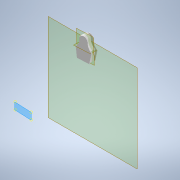
# Autodesk Inventor part: sprocket7_mk2_tips
Saved by Autodesk Inventor 2020 (Build 240168000, 168)
## iProperties
Created: 2019-08-05
Part Number: sprocket7_mk2_tips
Material: Generic
Document SubType Name: Modeling
Designer: erwin
Density: 1 g/cm^3
Appearance: Default
Author: erwin
Autodesk Inventor part; units mm, degrees
ref_plane "YZ Plane" through (0, 0, 0) normal (1, 0, 0) x (0, 1, 0)
ref_plane "XZ Plane" through (0, 0, 0) normal (0, 1, 0) x (-1, 0, 0)
ref_plane "XY Plane" through (0, 0, 0) normal (0, 0, 1) x (1, 0, 0)
ref_plane "Work Plane1" through (6.098, -2.6064, -12) normal (0, 0, -1) x (-1, 0, 0)
sketch "Sketch1" plane through (6.098, -2.6064, -12) normal (0, 0, -1) x (-1, 0, 0)
  circle A0 centre (7.1179, -1.5237) radius 10.75 construction
  arc A1 (21.9255, 105.301) -> (1.9456, 106.1983) centre (11.9355, 105.7496) ccw construction
  line L0 (-93.2965, -27.178) -> (-90.244, -26.8147) projected
  line L1 (-90.244, -26.8147) -> (-85.3551, -26.6226) projected
  line L2 (-85.3551, -26.6226) -> (-80.6041, -27.7915) projected
  line L3 (-80.6041, -27.7915) -> (-76.3624, -30.2299) projected
  line L4 (-76.3624, -30.2299) -> (-72.9614, -33.7473) projected
  line L5 (-72.9614, -33.7473) -> (-48.2745, -67.726) projected
  line L6 (-48.2745, -67.726) -> (-45.9802, -72.0474) projected
  line L7 (-45.9802, -72.0474) -> (-44.9719, -76.835) projected
  line L8 (-44.9719, -76.835) -> (-45.3284, -81.7147) projected
  line L9 (-45.3284, -81.7147) -> (-47.0218, -86.3049) projected
  line L10 (-47.0218, -86.3049) -> (-48.3106, -89.0958) projected
  line L11 (-48.3106, -89.0958) -> (-48.988, -90.8804) projected
  line L12 (-48.988, -90.8804) -> (-49.1805, -92.7796) projected
  line L13 (-49.1805, -92.7796) -> (-48.8748, -94.6639) projected
  line L14 (-48.8748, -94.6639) -> (-48.0919, -96.4049) projected
  line L15 (-48.0919, -96.4049) -> (-46.885, -97.8839) projected
  line L16 (-46.885, -97.8839) -> (-45.3365, -99.0002) projected
  line L17 (-45.3365, -99.0002) -> (-43.5518, -99.6776) projected
  line L18 (-43.5518, -99.6776) -> (-41.6526, -99.87) projected
  line L19 (-41.6526, -99.87) -> (-39.7683, -99.5643) projected
  line L20 (-39.7683, -99.5643) -> (-38.0273, -98.7814) projected
  line L21 (-38.0273, -98.7814) -> (-36.5483, -97.5745) projected
  line L22 (-36.5483, -97.5745) -> (-35.4321, -96.026) projected
  line L23 (-35.4321, -96.026) -> (-33.8129, -93.4129) projected
  line L24 (-33.8129, -93.4129) -> (-30.9149, -89.4709) projected
  line L25 (-30.9149, -89.4709) -> (-27.0389, -86.4852) projected
  line L26 (-27.0389, -86.4852) -> (-22.4878, -84.6892) projected
  line L27 (-22.4878, -84.6892) -> (-17.6173, -84.2233) projected
  line L28 (-17.6173, -84.2233) -> (24.3404, -86.1076) projected
  line L29 (24.3404, -86.1076) -> (29.1494, -87.0082) projected
  line L30 (29.1494, -87.0082) -> (33.5212, -89.2049) projected
  line L31 (33.5212, -89.2049) -> (37.114, -92.5261) projected
  line L32 (37.114, -92.5261) -> (39.647, -96.712) projected
  line L33 (39.647, -96.712) -> (41.0254, -99.4597) projected
  line L34 (41.0254, -99.4597) -> (41.9983, -101.1021) projected
  line L35 (41.9983, -101.1021) -> (43.3632, -102.4367) projected
  line L36 (43.3632, -102.4367) -> (45.027, -103.3725) projected
  line L37 (45.027, -103.3725) -> (46.8763, -103.8459) projected
  line L38 (46.8763, -103.8459) -> (48.7851, -103.8244) projected
  line L39 (48.7851, -103.8244) -> (50.6233, -103.3097) projected
  line L40 (50.6233, -103.3097) -> (52.2657, -102.3368) projected
  line L41 (52.2657, -102.3368) -> (53.6003, -100.9719) projected
  line L42 (53.6003, -100.9719) -> (54.5361, -99.3081) projected
  line L43 (54.5361, -99.3081) -> (55.0095, -97.4588) projected
  line L44 (55.0095, -97.4588) -> (54.988, -95.55) projected
  line L45 (54.988, -95.55) -> (54.4733, -93.7118) projected
  line L46 (54.4733, -93.7118) -> (53.4399, -90.8167) projected
  line L47 (53.4399, -90.8167) -> (52.1647, -86.0931) projected
  line L48 (52.1647, -86.0931) -> (52.2471, -81.2011) projected
  line L49 (52.2471, -81.2011) -> (53.6805, -76.5231) projected
  line L50 (53.6805, -76.5231) -> (56.3529, -72.4248) projected
  line L51 (56.3529, -72.4248) -> (83.9863, -40.7958) projected
  line L52 (83.9863, -40.7958) -> (87.6888, -37.5974) projected
  line L53 (87.6888, -37.5974) -> (92.1321, -35.5491) projected
  line L54 (92.1321, -35.5491) -> (96.9687, -34.8108) projected
  line L55 (96.9687, -34.8108) -> (101.8207, -35.4404) projected
  line L56 (101.8207, -35.4404) -> (104.8283, -36.0758) projected
  line L57 (104.8283, -36.0758) -> (106.719, -36.3391) projected
  line L58 (106.719, -36.3391) -> (108.6134, -36.1041) projected
  line L59 (108.6134, -36.1041) -> (110.3825, -35.3868) projected
  line L60 (110.3825, -35.3868) -> (111.9056, -34.2361) projected
  line L61 (111.9056, -34.2361) -> (113.0789, -32.7304) projected
  line L62 (113.0789, -32.7304) -> (113.8226, -30.9723) projected
  line L63 (113.8226, -30.9723) -> (114.0859, -29.0816) projected
  line L64 (114.0859, -29.0816) -> (113.8509, -27.1872) projected
  line L65 (113.8509, -27.1872) -> (113.1336, -25.4182) projected
  line L66 (113.1336, -25.4182) -> (111.9829, -23.8951) projected
  line L67 (111.9829, -23.8951) -> (110.4772, -22.7217) projected
  line L68 (110.4772, -22.7217) -> (108.7191, -21.978) projected
  line L69 (108.7191, -21.978) -> (105.8112, -20.9809) projected
  line L70 (105.8112, -20.9809) -> (101.3232, -19.0328) projected
  line L71 (101.3232, -19.0328) -> (97.5498, -15.9183) projected
  line L72 (97.5498, -15.9183) -> (94.7861, -11.881) projected
  line L73 (94.7861, -11.881) -> (93.2481, -7.2363) projected
  line L74 (93.2481, -7.2363) -> (85.7487, 34.0887) projected
  line L75 (85.7487, 34.0887) -> (85.5567, 38.9776) projected
  line L76 (85.5567, 38.9776) -> (86.7255, 43.7286) projected
  line L77 (86.7255, 43.7286) -> (89.1639, 47.9703) projected
  line L78 (89.1639, 47.9703) -> (92.6813, 51.3713) projected
  line L79 (92.6813, 51.3713) -> (95.0533, 53.3265) projected
  line L80 (95.0533, 53.3265) -> (96.438, 54.6406) projected
  line L81 (96.438, 54.6406) -> (97.4354, 56.2682) projected
  line L82 (97.4354, 56.2682) -> (97.9776, 58.0985) projected
  line L83 (97.9776, 58.0985) -> (98.0276, 60.0068) projected
  line L84 (98.0276, 60.0068) -> (97.5819, 61.8629) projected
  line L85 (97.5819, 61.8629) -> (96.6711, 63.5405) projected
  line L86 (96.6711, 63.5405) -> (95.357, 64.9252) projected
  line L87 (95.357, 64.9252) -> (93.7294, 65.9226) projected
  line L88 (93.7294, 65.9226) -> (91.8991, 66.4648) projected
  line L89 (91.8991, 66.4648) -> (89.9908, 66.5148) projected
  line L90 (89.9908, 66.5148) -> (88.1347, 66.0691) projected
  line L91 (88.1347, 66.0691) -> (86.4571, 65.1583) projected
  line L92 (86.4571, 65.1583) -> (83.8645, 63.5065) projected
  line L93 (83.8645, 63.5065) -> (79.5431, 61.2122) projected
  line L94 (79.5431, 61.2122) -> (74.7554, 60.204) projected
  line L95 (74.7554, 60.204) -> (69.8758, 60.5605) projected
  line L96 (69.8758, 60.5605) -> (65.2855, 62.2539) projected
  line L97 (65.2855, 62.2539) -> (28.3005, 82.1564) projected
  line L98 (28.3005, 82.1564) -> (24.3585, 85.0544) projected
  line L99 (24.3585, 85.0544) -> (21.3728, 88.9304) projected
  line L100 (21.3728, 88.9304) -> (19.5768, 93.4815) construction
  line L101 (19.5768, 93.4815) -> (19.1109, 98.3519) projected
  line L102 (19.1109, 98.3519) -> (19.0611, 101.4256) projected
  line L103 (19.0611, 101.4256) -> (18.8971, 103.3274) projected
  line L104 (18.8971, 103.3274) -> (18.2465, 105.1221) projected
  line L105 (18.2465, 105.1221) -> (17.1535, 106.6871) projected
  line L106 (17.1535, 106.6871) -> (15.6927, 107.916) projected
  line L107 (15.6927, 107.916) -> (13.9636, 108.7249) projected
  line L108 (13.9636, 108.7249) -> (12.0841, 109.0587) projected
  line L109 (12.0841, 109.0587) -> (10.1823, 108.8947) projected
  line L110 (10.1823, 108.8947) -> (8.3877, 108.244) projected
  line L111 (8.3877, 108.244) -> (6.8226, 107.1511) projected
  line L112 (6.8226, 107.1511) -> (5.5937, 105.6903) projected
  line L113 (5.5937, 105.6903) -> (4.7848, 103.9612) projected
  line L114 (4.7848, 103.9612) -> (4.451, 102.0817) projected
  line L115 (4.451, 102.0817) -> (4.126, 99.0249) projected
  line L116 (4.126, 99.0249) -> (3.2253, 94.2159) projected
  line L117 (3.2253, 94.2159) -> (1.0286, 89.8441) construction
  line L118 (1.0286, 89.8441) -> (-2.2925, 86.2513) projected
  line L119 (-2.2925, 86.2513) -> (-6.4785, 83.7183) projected
  line L120 (-6.4785, 83.7183) -> (-45.0987, 67.2113) projected
  line L121 (-45.0987, 67.2113) -> (-49.8222, 65.9361) projected
  line L122 (-49.8222, 65.9361) -> (-54.7142, 66.0184) projected
  line L123 (-54.7142, 66.0184) -> (-59.3922, 67.4518) projected
  line L124 (-59.3922, 67.4518) -> (-63.4905, 70.1242) projected
  line L125 (-63.4905, 70.1242) -> (-65.9246, 72.0017) projected
  line L126 (-65.9246, 72.0017) -> (-67.5138, 73.0593) projected
  line L127 (-67.5138, 73.0593) -> (-69.3226, 73.6695) projected
  line L128 (-69.3226, 73.6695) -> (-71.2276, 73.7908) projected
  line L129 (-71.2276, 73.7908) -> (-73.0992, 73.4149) projected
  line L130 (-73.0992, 73.4149) -> (-74.8096, 72.5674) projected
  line L131 (-74.8096, 72.5674) -> (-76.2425, 71.3061) projected
  line L132 (-76.2425, 71.3061) -> (-77.3001, 69.7169) projected
  line L133 (-77.3001, 69.7169) -> (-77.9103, 67.9081) projected
  line L134 (-77.9103, 67.9081) -> (-78.0316, 66.0031) projected
  line L135 (-78.0316, 66.0031) -> (-77.6557, 64.1315) projected
  line L136 (-77.6557, 64.1315) -> (-76.8082, 62.4211) projected
  line L137 (-76.8082, 62.4211) -> (-75.5468, 60.9882) projected
  line L138 (-75.5468, 60.9882) -> (-73.3596, 58.8282) projected
  line L139 (-73.3596, 58.8282) -> (-70.1612, 55.1256) projected
  line L140 (-70.1612, 55.1256) -> (-68.1129, 50.6824) projected
  line L141 (-68.1129, 50.6824) -> (-67.3746, 45.8458) projected
  line L142 (-67.3746, 45.8458) -> (-68.0042, 40.9938) projected
  line L143 (-68.0042, 40.9938) -> (-79.1777, 0.5073) projected
  line L144 (-79.1777, 0.5073) -> (-81.1259, -3.9807) projected
  line L145 (-81.1259, -3.9807) -> (-84.2403, -7.7541) projected
  line L146 (-84.2403, -7.7541) -> (-88.2777, -10.5178) projected
  line L147 (-88.2777, -10.5178) -> (-92.9223, -12.0558) projected
  line L148 (-92.9223, -12.0558) -> (-95.9078, -12.7882) projected
  line L149 (-95.9078, -12.7882) -> (-97.7255, -13.3713) projected
  line L150 (-97.7255, -13.3713) -> (-99.3304, -14.405) projected
  line L151 (-99.3304, -14.405) -> (-100.613, -15.8188) projected
  line L152 (-100.613, -15.8188) -> (-101.486, -17.5164) projected
  line L153 (-101.486, -17.5164) -> (-101.8898, -19.3821) projected
  line L154 (-101.8898, -19.3821) -> (-101.7971, -21.2888) projected
  line L155 (-101.7971, -21.2888) -> (-101.214, -23.1065) projected
  line L156 (-101.214, -23.1065) -> (-100.1803, -24.7113) projected
  line L157 (-100.1803, -24.7113) -> (-98.7665, -25.9939) projected
  line L158 (-98.7665, -25.9939) -> (-97.0689, -26.8669) projected
  line L159 (-97.0689, -26.8669) -> (-95.2031, -27.2708) projected
  line L160 (-95.2031, -27.2708) -> (-93.2965, -27.178) projected
  circle A2 centre (7.1179, -1.5237) radius 10.75 projected
  circle A3 centre (11.7561, 101.7537) radius 7.2498
  line L161 (-3.033, 62.3775) -> (22.956, 61.2104) projected
  line L162 (-4.0017, 85.217) -> (-3.033, 62.3775) projected
  line L163 (22.956, 61.2104) -> (25.9681, 83.8711) projected
  arc A4 (-4.0017, 85.217) -> (4.5067, 101.6713) centre (-15.2247, 101.4473) ccw
  line L164 (11.7561, 101.7537) -> (7.1179, -1.5237) construction
  arc A5 (18.9689, 101.0219) -> (25.9681, 83.8711) centre (38.6007, 99.03) ccw
  point P0 (6.098, 2.6064)
  point P1 (11.3971, 93.7617)
  point P2 (21.2089, 89.3457)
  point P3 (1.229, 90.2429)
  point P4 (19.0059, 101.7435)
  point P5 (18.9689, 101.0219)
  constraints: 8 point on circle, 5 tangent, 4 centre point, 2 end point, 2 point on line, 2 symmetric about line, 1 other
extrude "Extrusion1" add sketch "Sketch1" against normal blind 12 contours A4 A3 A5 L163 L161 L162 | A3
sketch "Sketch2" plane through (6.098, -2.6064, 0) normal (0, 0, 1) x (-1, 0, 0)
  line L0 (1.229, 90.2429) -> (21.2089, 89.3456) projected
  line L1 (1.229, 90.2429) -> (0.8688, 82.2225) projected
  arc A0 (0.8688, 82.2225) -> (20.8487, 81.3252) centre (10.8588, 81.7738) ccw projected
  line L2 (20.8487, 81.3252) -> (21.2089, 89.3456) projected
  arc A1 (-1.9524, 82.3492) -> (23.67, 81.1985) centre (10.8588, 81.7738) ccw
  line L3 (-1.9524, 82.3492) -> (-1.4655, 93.1909)
  line L4 (-1.4655, 93.1909) -> (24.1569, 92.0402)
  line L5 (24.1569, 92.0402) -> (23.67, 81.1985)
  circle A2 centre (10.8588, 81.7738) radius 12.8241
  circle A3 centre (10.8588, 81.7738) radius 7.8241
  line L6 (20.8487, 81.3252) -> (21.2089, 89.3456) projected
  arc A4 (21.2089, 89.3456) -> (18.6806, 81.5855) centre (32.905, 81.2431) ccw
  line L7 (10.8588, 81.7738) -> (12.0813, 108.9962) construction
  arc A5 (19.0059, 101.7435) -> (4.5341, 102.3888) centre (11.7561, 101.7537) ccw projected
  arc A6 (3.0515, 82.2874) -> (1.229, 90.2429) centre (-11.1463, 83.2214) ccw
  point P0 (6.098, -2.6064)
  point P1 (1.2053, 89.7149)
  point P2 (-1.9524, 82.3492)
  point P3 (21.1852, 88.8176)
  point P4 (1.229, 90.2429)
  point P5 (1.229, 90.2429)
  point P6 (1.0296, 90.0106)
  point P7 (3.0515, 82.2874)
  point P8 (1.229, 90.2429)
  dimension "d10" = 5
  constraints: 9 point on circle, 8 end point, 4 centre point, 3 symmetric about line, 2 coincident, 8 other
sketch "Sketch3" plane through (-4.7607, 79.1674, -11) normal (0, 0, 1) x (0.9989931, 0.0448647, 0)
  arc A0 (-7.8224, 0.1628) -> (7.8224, 0.1628) centre (0, 0) ccw projected
  arc A1 (-7.8224, 0.1628) -> (-10, 8.0286) centre (-22.0479, 0.4589) ccw projected
  arc A2 (-10, 8.0286) -> (10, 8.0286) centre (0, 0) ccw projected
  arc A3 (10, 8.0286) -> (7.8224, 0.1628) centre (22.0479, 0.4589) ccw projected
  arc A4 (-7.9795, 8.0286) -> (-5.2449, 20.5755) centre (-42.9142, 22.2142) ccw projected
  line L0 (-7.9795, 8.0286) -> (7.9795, 8.0286) projected
  arc A5 (5.245, 20.5722) -> (7.9795, 8.0286) centre (42.9142, 22.2142) ccw projected
  arc A6 (5.245, 20.5722) -> (-5.2449, 20.5755) centre (0, 20.3473) ccw projected
  line L1 (0, 20.3473) -> (0, 0) construction
  line L2 (0, 0) -> (0, -15) construction
  line L3 (-12.8241, 0) -> (-12.8241, -15) construction
  line L4 (12.8241, -15) -> (12.8241, 0) construction
  arc A7 (12.8241, 0) -> (-12.8241, 0) centre (0, 0) ccw construction
  arc A8 (-12.8241, -15) -> (12.8241, -15) centre (0, -15) ccw construction
  arc A9 (-10, 8.0286) -> (10, 8.0286) centre (0, 0) ccw construction
  arc A10 (-7.8224, 0.1628) -> (7.8224, 0.1628) centre (0, 0) ccw construction
  line L5 (0, 0) -> (0, -18.52) construction
  line L6 (-6, -14.0249) -> (-6, -18.52) construction
  line L7 (6, -18.52) -> (6, -14.0249) construction
  arc A11 (6, 0) -> (-6, 0) centre (0, 0) ccw construction
  arc A12 (-6, -18.52) -> (6, -18.52) centre (0, -18.52) ccw construction
  line L8 (6, -18.52) -> (6, -11.3339)
  line L9 (-6, -18.52) -> (-6, -11.3339)
  arc A13 (7.9143, -10.0907) -> (-7.9143, -10.0907) centre (0, 0) ccw
  arc A14 (-6, -18.52) -> (6, -18.52) centre (0, -18.52) ccw
  arc A15 (7.9143, -10.0907) -> (6, -14.0249) centre (11, -14.0249) ccw
  arc A16 (-6, -14.0249) -> (-7.9143, -10.0907) centre (-11, -14.0249) ccw
  point P0 (1.2041, -79.3013)
  point P1 (0, -7.5)
  point P2 (0, -9.26)
  point P3 (6, -14.0249)
  point P4 (7.9143, -10.0907)
  point P5 (-7.9143, -10.0907)
  point P6 (-6, -14.0249)
  dimension "d17" = 15
  dimension "d18" = 12
  dimension "d19" = 5
  constraints: 22 end point, 21 point on circle, 12 tangent, 8 centre point, 5 point on line, 2 coincident, 2 equal radius, 2 midpoint, 2 parallel, 1 collinear, 1 vertical
  measures "d17" distance of L1.end L2.end
  measures "d18" diameter of A12
  measures "d19" radius of A15
sketch "Sketch4" plane through (-4.7607, 79.1674, -11) normal (0, 0, 1) x (0.9989931, 0.0448647, 0)
  arc A0 (-6, -18.52) -> (6, -18.52) centre (0, -18.52) ccw projected
  point P0 (1.2041, -79.3013)
  constraints: 1 coincident
move faces "Move1" translate (0, 0, 1) faces at (-8.1018, 67.7151, 0)
move faces "Move2" translate (0, 0, -1) faces at (-8.1018, 67.7151, -12)
sketch "Sketch5" plane through (-5.658, 99.1472, 1) normal (0, 0, 1) x (0.9989931, 0.0448648, 0)
  arc A0 (11.348, -0.4075) -> (-3.1288, -0.4075) centre (4.1096, 0) ccw
  arc A1 (-12.1986, -18.1402) -> (-3.1288, -0.4075) centre (-22.8302, -1.5165) ccw
  line L0 (-4.7883, -40) -> (13.0076, -40)
  arc A2 (11.348, -0.4075) -> (20.4179, -18.1402) centre (31.0495, -1.5165) ccw
  line L1 (-6.3413, -40) -> (-12.6076, -16.6138)
  arc A3 (-12.6076, -16.6138) -> (-4.6264, -0.4918) centre (-22.8302, -1.5165) ccw
  arc A4 (12.8457, -0.4918) -> (-4.6264, -0.4918) centre (4.1096, 0) ccw
  arc A5 (12.8457, -0.4918) -> (20.8268, -16.6138) centre (31.0495, -1.5165) ccw
  line L2 (20.8268, -16.6138) -> (14.5605, -40)
  line L3 (-10.8904, -17.227) -> (-4.7883, -40)
  line L4 (-4.7883, -40) -> (-6.3413, -40)
  line L5 (-4.7883, -40) -> (13.0076, -40)
  line L6 (13.0076, -40) -> (14.5605, -40)
  line L7 (13.0076, -40) -> (15, -17.227) projected
  point P0 (1.2041, -99.3012)
  point P1 (-10.8904, -17.227)
  constraints: 14 end point, 10 point on circle, 6 centre point, 2 point on line, 5 other
extrude "Extrusion4" add sketch "Sketch5" against normal blind 1
ref_plane "Work Plane4" through (-5.658, 99.1472, -6) normal (0, 0, -1) x (-0.9989931, -0.0448648, 0)
mirror "Mirror2" about plane through (-5.658, 99.1472, -6) normal (0, 0, -1) of "Extrusion4"
ref_plane "Work Plane5" through (-21.136, 80.2937, 1) normal (0.0448649, -0.9989931, 0) x (0, 0, -1)
split "Split2" [suppressed]
feature "FaceDraft3" [suppressed]
feature "FaceDraft4" [suppressed]
fillet "Fillet2" radius 2 4 edges at (-11.4181, 103.5497, -13) (-14.2329, 88.9677, -13) (-11.4181, 103.5497, 1) (-14.2329, 88.9677, 1)
sketch "Sketch6" plane through (10.5709, 59.8357, -13) normal (0, 0, -1) x (-0.9989931, -0.0448648, 0)
  line L0 (-15.5913, 20.1715) -> (-10.7459, 20.1715) construction
  line L1 (-10.7459, 20.1715) -> (-10.7459, 15.3261) construction
  line L2 (-10.7459, 15.3261) -> (-15.5913, 15.3261) construction
  line L3 (-15.5913, 15.3261) -> (-15.5913, 20.1715) construction
  line L4 (-25.2062, 21.8598) -> (7.4102, 21.8598) projected
  point P0 (13.2447, -59.3012)
  constraints: 3 equal length, 1 parallel, 2 other
emboss "Emboss1" [suppressed]
body "Solid1"
body "Solid2"
body "Solid3"
body "Solid4"
body "Solid5"
